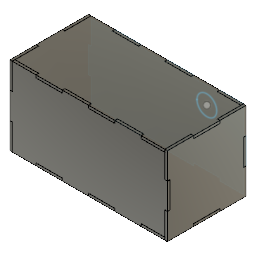
box 4 whole v4 (Autodesk Fusion 360 design; units mm, degrees)
Autodesk Fusion 360 part; units mm, degrees
sketch "Sketch1" plane through (0, 0, 0) normal (0, 0, 1) x (1, 0, 0)
  line L0 (0, 0) -> (120, 0)
  line L1 (120, 0) -> (120, 60)
  line L2 (120, 60) -> (0, 60)
  line L3 (0, 60) -> (0, 0)
  line L4 (0, 60) -> (20, 60)
  line L5 (20, 60) -> (20, 58)
  line L6 (20, 58) -> (0, 58)
  line L7 (0, 58) -> (0, 60)
  line L8 (20, 60) -> (40, 60)
  line L9 (40, 60) -> (40, 58)
  line L10 (40, 58) -> (20, 58)
  line L11 (20, 58) -> (20, 60)
  line L12 (40, 60) -> (60, 60)
  line L13 (60, 60) -> (60, 58)
  line L14 (60, 58) -> (40, 58)
  line L15 (40, 58) -> (40, 60)
  line L16 (60, 60) -> (80, 60)
  line L17 (80, 60) -> (80, 58)
  line L18 (80, 58) -> (60, 58)
  line L19 (60, 58) -> (60, 60)
  line L20 (80, 60) -> (100, 60)
  line L21 (100, 60) -> (100, 58)
  line L22 (100, 58) -> (80, 58)
  line L23 (80, 58) -> (80, 60)
  line L24 (100, 60) -> (120, 60)
  line L25 (120, 60) -> (120, 58)
  line L26 (120, 58) -> (100, 58)
  line L27 (100, 58) -> (100, 60)
  line L28 (120, 60) -> (118, 60)
  line L29 (118, 60) -> (118, 40)
  line L30 (118, 40) -> (120, 40)
  line L31 (120, 40) -> (120, 60)
  line L32 (118, 40) -> (120, 40)
  line L33 (120, 40) -> (120, 20)
  line L34 (120, 20) -> (118, 20)
  line L35 (118, 20) -> (118, 40)
  line L36 (120, 20) -> (118, 20)
  line L37 (118, 20) -> (118, 0)
  line L38 (118, 0) -> (120, 0)
  line L39 (120, 0) -> (120, 20)
  line L40 (120, 0) -> (100, 0)
  line L41 (100, 0) -> (100, 2)
  line L42 (100, 2) -> (120, 2)
  line L43 (120, 2) -> (120, 0)
  line L44 (100, 2) -> (80, 2)
  line L45 (80, 2) -> (80, 0)
  line L46 (80, 0) -> (100, 0)
  line L47 (100, 0) -> (100, 2)
  line L48 (80, 2) -> (60, 2)
  line L49 (60, 2) -> (60, 0)
  line L50 (60, 0) -> (80, 0)
  line L51 (80, 0) -> (80, 2)
  line L52 (60, 2) -> (40, 2)
  line L53 (40, 2) -> (40, 0)
  line L54 (40, 0) -> (60, 0)
  line L55 (60, 0) -> (60, 2)
  line L56 (40, 2) -> (20, 2)
  line L57 (20, 2) -> (20, 0)
  line L58 (20, 0) -> (40, 0)
  line L59 (40, 0) -> (40, 2)
  line L60 (20, 2) -> (0, 2)
  line L61 (0, 2) -> (0, 0)
  line L62 (0, 0) -> (20, 0)
  line L63 (20, 0) -> (20, 2)
  line L64 (0, 0) -> (2, 0)
  line L65 (2, 0) -> (2, 20)
  line L66 (2, 20) -> (0, 20)
  line L67 (0, 20) -> (0, 0)
  line L68 (0, 20) -> (2, 20)
  line L69 (2, 20) -> (2, 40)
  line L70 (2, 40) -> (0, 40)
  line L71 (0, 40) -> (0, 20)
  line L72 (0, 40) -> (2, 40)
  line L73 (2, 40) -> (2, 60)
  line L74 (2, 60) -> (0, 60)
  line L75 (0, 60) -> (0, 40)
  dimension "d1" = 120
  dimension "d2" = 60
  dimension "d3" = 20
  dimension "d4" = 2
  dimension "d5" = 20
  dimension "d6" = 2
  dimension "d7" = 20
  dimension "d8" = 2
  dimension "d9" = 20
  dimension "d10" = 2
  dimension "d11" = 20
  dimension "d12" = 2
  dimension "d13" = 20
  dimension "d14" = 2
  dimension "d15" = 2
  dimension "d16" = 20
  dimension "d17" = 2
  dimension "d18" = 20
  dimension "d19" = 2
  dimension "d20" = 20
  dimension "d21" = 20
  dimension "d22" = 2
  dimension "d23" = 20
  dimension "d24" = 2
  dimension "d25" = 20
  dimension "d26" = 2
  dimension "d27" = 20
  dimension "d28" = 2
  dimension "d29" = 20
  dimension "d30" = 2
  dimension "d31" = 20
  dimension "d32" = 2
  dimension "d33" = 2
  dimension "d34" = 20
  dimension "d35" = 2
  dimension "d36" = 20
  dimension "d37" = 2
  dimension "d38" = 20
  constraint horizontal L0
  constraint vertical L1
  constraint horizontal L2
  constraint vertical L3
  constraint coincident L0.start L3.end
  constraint horizontal L4
  constraint vertical L5
  constraint horizontal L6
  constraint vertical L7
  constraint horizontal L8
  constraint vertical L9
  constraint horizontal L10
  constraint vertical L11
  constraint horizontal L12
  constraint vertical L13
  constraint horizontal L14
  constraint vertical L15
  constraint horizontal L16
  constraint vertical L17
  constraint horizontal L18
  constraint vertical L19
  constraint horizontal L20
  constraint vertical L21
  constraint horizontal L22
  constraint vertical L23
  constraint horizontal L24
  constraint vertical L25
  constraint horizontal L26
  constraint vertical L27
  constraint horizontal L28
  constraint vertical L29
  constraint horizontal L30
  constraint vertical L31
  constraint horizontal L32
  constraint vertical L33
  constraint horizontal L34
  constraint vertical L35
  constraint horizontal L36
  constraint vertical L37
  constraint horizontal L38
  constraint vertical L39
  constraint horizontal L40
  constraint vertical L41
  constraint horizontal L42
  constraint vertical L43
  constraint horizontal L44
  constraint vertical L45
  constraint horizontal L46
  constraint vertical L47
  constraint horizontal L48
  constraint vertical L49
  constraint horizontal L50
  constraint vertical L51
  constraint horizontal L52
  constraint vertical L53
  constraint horizontal L54
  constraint vertical L55
  constraint horizontal L56
  constraint vertical L57
  constraint horizontal L58
  constraint vertical L59
  constraint horizontal L60
  constraint vertical L61
  constraint horizontal L62
  constraint vertical L63
  constraint horizontal L64
  constraint vertical L65
  constraint horizontal L66
  constraint vertical L67
  constraint horizontal L68
  constraint vertical L69
  constraint horizontal L70
  constraint vertical L71
  constraint horizontal L72
  constraint vertical L73
  constraint horizontal L74
  constraint vertical L75
  measures "d1" distance of L0.start L0.end
  measures "d2" distance of L0.start L2.end
  measures "d3" distance of L2.end L4.end
  measures "d4" distance of L2.end L6.end
  measures "d5" distance of L4.end L8.end
  measures "d6" distance of L4.end L5.end
  measures "d7" distance of L8.end L12.end
  measures "d8" distance of L8.end L9.end
  measures "d9" distance of L12.end L16.end
  measures "d10" distance of L12.end L13.end
  measures "d11" distance of L16.end L20.end
  measures "d12" distance of L16.end L17.end
  measures "d13" distance of L20.end L1.end
  measures "d14" distance of L20.end L21.end
  measures "d15" distance of L1.end L28.end
  measures "d16" distance of L1.end L30.end
  measures "d17" distance of L29.end L30.end
  measures "d18" distance of L29.end L34.end
  measures "d19" distance of L33.end L34.end
  measures "d20" distance of L33.end L0.end
  measures "d21" distance of L0.end L40.end
  measures "d22" distance of L0.end L42.end
  measures "d23" distance of L41.end L44.end
  measures "d24" distance of L41.end L40.end
  measures "d25" distance of L44.end L48.end
  measures "d26" distance of L44.end L45.end
  measures "d27" distance of L48.end L52.end
  measures "d28" distance of L48.end L49.end
  measures "d29" distance of L52.end L56.end
  measures "d30" distance of L52.end L53.end
  measures "d31" distance of L56.end L60.end
  measures "d32" distance of L56.end L57.end
  measures "d33" distance of L0.start L64.end
  measures "d34" distance of L0.start L66.end
  measures "d35" distance of L66.end L65.end
  measures "d36" distance of L66.end L70.end
  measures "d37" distance of L70.end L69.end
  measures "d38" distance of L70.end L2.end
extrude "Extrude1" add sketch "Sketch1" along normal blind 2 contours L0 L53 L56 L57 L58 L59 L63 | L6 L10 L14 L18 L22 L26 L29 L35 L37 L42 L44 L48 L52 L56 L60 L65 L69 L73 | L3 L66 L68 L69 L70 L71 L72 | L0 L45 L48 L49 L50 L51 L55 | L2 L4 L5 L6 L11 L73 | L0 L37 L40 L41 L42 L47 | L2 L9 L12 L13 L14 L15 L19 | L1 L30 L32 L33 L34 L35 L36 | L2 L17 L20 L21 L22 L23 L27 makes body 1
sketch "Sketch2" plane through (0, 0, 0) normal (1, 0, 0) x (0, 1, 0)
  line L0 (0, 0) -> (60, 0)
  line L1 (60, 0) -> (60, 60)
  line L2 (60, 60) -> (0, 60)
  line L3 (0, 60) -> (0, 0)
  line L4 (60, 0) -> (40, 0)
  line L5 (40, 0) -> (40, 2)
  line L6 (40, 2) -> (60, 2)
  line L7 (60, 2) -> (60, 0)
  line L8 (0, 0) -> (20, 0)
  line L9 (20, 0) -> (20, 2)
  line L10 (20, 2) -> (0, 2)
  line L11 (0, 2) -> (0, 0)
  line L12 (0, 60) -> (2, 60)
  line L13 (2, 60) -> (2, 40)
  line L14 (2, 40) -> (0, 40)
  line L15 (0, 40) -> (0, 60)
  line L16 (2, 40) -> (0, 40)
  line L17 (0, 40) -> (0, 20)
  line L18 (0, 20) -> (2, 20)
  line L19 (2, 20) -> (2, 40)
  line L20 (0, 20) -> (2, 20)
  line L21 (2, 20) -> (2, 0)
  line L22 (2, 0) -> (0, 0)
  line L23 (0, 0) -> (0, 20)
  line L24 (60, 60) -> (58, 60)
  line L25 (58, 60) -> (58, 40)
  line L26 (58, 40) -> (60, 40)
  line L27 (60, 40) -> (60, 60)
  line L28 (58, 40) -> (60, 40)
  line L29 (60, 40) -> (60, 20)
  line L30 (60, 20) -> (58, 20)
  line L31 (58, 20) -> (58, 40)
  line L32 (60, 20.0791) -> (58, 20.0791)
  line L33 (58, 20.0791) -> (58, 0)
  line L34 (58, 0) -> (60, 0)
  line L35 (60, 0) -> (60, 20.0791)
  line L36 (60, 60) -> (40, 60)
  line L37 (40, 60) -> (40, 58)
  line L38 (40, 58) -> (60, 58)
  line L39 (60, 58) -> (60, 60)
  line L40 (40, 60) -> (20, 60)
  line L41 (20, 60) -> (20, 58)
  line L42 (20, 58) -> (40, 58)
  line L43 (40, 58) -> (40, 60)
  line L44 (20, 60) -> (0, 60)
  line L45 (0, 60) -> (0, 58)
  line L46 (0, 58) -> (20, 58)
  line L47 (20, 58) -> (20, 60)
  line L48 (40, 2) -> (20, 2)
  line L49 (20, 2) -> (20, 0)
  line L50 (20, 0) -> (40, 0)
  line L51 (40, 0) -> (40, 2)
  dimension "d41" = 60
  dimension "d42" = 60
  constraint horizontal L0
  constraint vertical L1
  constraint horizontal L2
  constraint vertical L3
  constraint coincident L0.start L3.end
  constraint horizontal L4
  constraint vertical L5
  constraint horizontal L6
  constraint vertical L7
  constraint horizontal L8
  constraint vertical L9
  constraint horizontal L10
  constraint vertical L11
  constraint horizontal L12
  constraint vertical L13
  constraint horizontal L14
  constraint vertical L15
  constraint horizontal L16
  constraint vertical L17
  constraint horizontal L18
  constraint vertical L19
  constraint coincident L3 L17.end
  constraint horizontal L20
  constraint vertical L21
  constraint horizontal L22
  constraint vertical L23
  constraint horizontal L24
  constraint vertical L25
  constraint horizontal L26
  constraint vertical L27
  constraint horizontal L28
  constraint vertical L29
  constraint horizontal L30
  constraint vertical L31
  constraint coincident L1 L29.end
  constraint horizontal L32
  constraint vertical L33
  constraint horizontal L34
  constraint vertical L35
  constraint coincident L4 L33.end
  constraint coincident L1 L32.start
  constraint horizontal L36
  constraint vertical L37
  constraint horizontal L38
  constraint vertical L39
  constraint horizontal L40
  constraint vertical L41
  constraint horizontal L42
  constraint vertical L43
  constraint horizontal L44
  constraint vertical L45
  constraint horizontal L46
  constraint vertical L47
  constraint coincident L15 L45.end
  constraint horizontal L48
  constraint vertical L49
  constraint horizontal L50
  constraint vertical L51
  measures "d41" distance of L0.start L0.end
  measures "d42" distance of L0.start L2.end
extrude "Extrude2" add sketch "Sketch2" along normal blind 2 separate body contours L0 L3 L8 L10 L11 L21 L22 L23 | L0 L8 L9 L10 L21 L49 | L3 L10 L18 L20 L21 L23 | L6 L10 L13 L19 L21 L25 L31 L33 L38 L42 L46 L48 | L0 L4 L5 L6 L33 L51 | L3 L13 L14 L15 L16 L46 | L0 L1 L4 L6 L7 L33 L34 L35 | L2 L3 L12 L13 L15 L44 L45 L46 | L1 L6 L30 L33 L35 | L2 L13 L41 L44 L46 L47 | L2 L25 L36 L37 L38 L43 | L1 L25 L26 L27 L28 L38 | L1 L2 L24 L25 L27 L36 L38 L39 makes body 2
ref_plane "WorkPlane1" through (61, 30, 30) normal (1, 0, 0) x (0, 0, -1)
mirror "Mirror1" about plane through (61, 30, 30) normal (1, 0, 0) of bodies 2 makes body 3
move_body "Move1" bodies 3 to x (1, 0, 0) y (0, 1, 0) z (0, 0, 1) at (-2, 0, 0)
ref_plane "WorkPlane2" through (60, 30, 31) normal (0, 0, 1) x (1, 0, 0)
mirror "Mirror2" about plane through (60, 30, 31) normal (0, 0, 1) of bodies 1 makes body 4
move_body "Move2" bodies 4 to x (1, 0, 0) y (0, 1, 0) z (0, 0, 1) at (0, 0, -2)
sketch "Sketch3" plane through (0, 0, 0) normal (0, 1, 0) x (1, 0, 0)
  line L0 (0, 0) -> (120, 0)
  line L1 (120, 0) -> (120, -60)
  line L2 (120, -60) -> (0, -60)
  line L3 (0, -60) -> (0, 0)
  line L4 (0, -60) -> (2, -60)
  line L5 (2, -60) -> (2, -40)
  line L6 (2, -40) -> (0, -40)
  line L7 (0, -40) -> (0, -60)
  line L8 (0, -40) -> (2, -40)
  line L9 (2, -40) -> (2, -20)
  line L10 (2, -20) -> (0, -20)
  line L11 (0, -20) -> (0, -40)
  line L12 (0, -20) -> (2, -20)
  line L13 (2, -20) -> (2, 0)
  line L14 (2, 0) -> (0, 0)
  line L15 (0, 0) -> (0, -20)
  line L16 (0, -60) -> (20, -60)
  line L17 (20, -60) -> (20, -58)
  line L18 (20, -58) -> (0, -58)
  line L19 (0, -58) -> (0, -60)
  line L20 (20, -60) -> (40, -60)
  line L21 (40, -60) -> (40, -58)
  line L22 (40, -58) -> (20, -58)
  line L23 (20, -58) -> (20, -60)
  line L24 (40, -60) -> (60, -60)
  line L25 (60, -60) -> (60, -58)
  line L26 (60, -58) -> (40, -58)
  line L27 (40, -58) -> (40, -60)
  line L28 (60, -60) -> (80, -60)
  line L29 (80, -60) -> (80, -58)
  line L30 (80, -58) -> (60, -58)
  line L31 (60, -58) -> (60, -60)
  line L32 (80, -60) -> (100, -60)
  line L33 (100, -60) -> (100, -58)
  line L34 (100, -58) -> (80, -58)
  line L35 (80, -58) -> (80, -60)
  line L36 (100, -60) -> (120, -60)
  line L37 (120, -60) -> (120, -58)
  line L38 (120, -58) -> (100, -58)
  line L39 (100, -58) -> (100, -60)
  line L40 (120, -60) -> (118, -60)
  line L41 (118, -60) -> (118, -40)
  line L42 (118, -40) -> (120, -40)
  line L43 (120, -40) -> (120, -60)
  line L44 (120, -40) -> (118, -40)
  line L45 (118, -40) -> (118, -20)
  line L46 (118, -20) -> (120, -20)
  line L47 (120, -20) -> (120, -40)
  line L48 (118, -20) -> (120, -20)
  line L49 (120, -20) -> (120, 0)
  line L50 (120, 0) -> (118, 0)
  line L51 (118, 0) -> (118, -20)
  line L52 (120, 0) -> (100, 0)
  line L53 (100, 0) -> (100, -2)
  line L54 (100, -2) -> (120, -2)
  line L55 (120, -2) -> (120, 0)
  line L56 (100, 0) -> (80, 0)
  line L57 (80, 0) -> (80, -2)
  line L58 (80, -2) -> (100, -2)
  line L59 (100, -2) -> (100, 0)
  line L60 (80, 0) -> (60, 0)
  line L61 (60, 0) -> (60, -2)
  line L62 (60, -2) -> (80, -2)
  line L63 (80, -2) -> (80, 0)
  line L64 (0, 0) -> (20, 0)
  line L65 (20, 0) -> (20, -2)
  line L66 (20, -2) -> (0, -2)
  line L67 (0, -2) -> (0, 0)
  line L68 (40, 0) -> (20, 0)
  line L69 (20, 0) -> (20, -2)
  line L70 (20, -2) -> (40, -2)
  line L71 (40, -2) -> (40, 0)
  line L72 (40, 0) -> (60, 0)
  line L73 (60, 0) -> (60, -2)
  line L74 (60, -2) -> (40, -2)
  line L75 (40, -2) -> (40, 0)
  constraint horizontal L0
  constraint vertical L1
  constraint horizontal L2
  constraint vertical L3
  constraint coincident L0.start L3.end
  constraint horizontal L4
  constraint vertical L5
  constraint horizontal L6
  constraint vertical L7
  constraint horizontal L8
  constraint vertical L9
  constraint horizontal L10
  constraint vertical L11
  constraint horizontal L12
  constraint vertical L13
  constraint horizontal L14
  constraint vertical L15
  constraint coincident L0 L13.end
  constraint horizontal L16
  constraint vertical L17
  constraint horizontal L18
  constraint vertical L19
  constraint horizontal L20
  constraint vertical L21
  constraint horizontal L22
  constraint vertical L23
  constraint horizontal L24
  constraint vertical L25
  constraint horizontal L26
  constraint vertical L27
  constraint horizontal L28
  constraint vertical L29
  constraint horizontal L30
  constraint vertical L31
  constraint horizontal L32
  constraint vertical L33
  constraint horizontal L34
  constraint vertical L35
  constraint horizontal L36
  constraint vertical L37
  constraint horizontal L38
  constraint vertical L39
  constraint coincident L1 L37.end
  constraint horizontal L40
  constraint vertical L41
  constraint horizontal L42
  constraint vertical L43
  constraint horizontal L44
  constraint vertical L45
  constraint horizontal L46
  constraint vertical L47
  constraint horizontal L48
  constraint vertical L49
  constraint horizontal L50
  constraint vertical L51
  constraint horizontal L52
  constraint vertical L53
  constraint horizontal L54
  constraint vertical L55
  constraint horizontal L56
  constraint vertical L57
  constraint horizontal L58
  constraint vertical L59
  constraint horizontal L60
  constraint vertical L61
  constraint horizontal L62
  constraint vertical L63
  constraint horizontal L64
  constraint vertical L65
  constraint horizontal L66
  constraint vertical L67
  constraint horizontal L68
  constraint vertical L69
  constraint horizontal L70
  constraint vertical L71
  constraint coincident L0 L68.start
  constraint horizontal L72
  constraint vertical L73
  constraint horizontal L74
  constraint vertical L75
extrude "Extrude3" add sketch "Sketch3" along normal blind 2 separate body contours L0 L13 L64 L65 L66 L69 | L5 L9 L13 L18 L22 L26 L30 L34 L38 L41 L45 L51 L54 L58 L62 L66 L70 L74 | L3 L6 L8 L9 L10 L11 L12 | L0 L61 L71 L72 L73 L74 L75 | L0 L53 L56 L57 L58 L59 L63 | L2 L5 L16 L17 L18 L23 | L2 L21 L24 L25 L26 L27 L31 | L1 L42 L44 L45 L46 L47 L48 | L2 L29 L32 L33 L34 L35 L39 makes body 5
sketch "Sketch4" plane through (0, 58, 0) normal (0, 1, 0) x (-1, 0, 0)
  line L0 (-118, 0) -> (-100, 0)
  line L1 (-100, 0) -> (-100, 2)
  line L2 (-100, 2) -> (-118, 2)
  line L3 (-118, 2) -> (-118, 0)
  line L4 (-120, 0) -> (0, 0)
  line L5 (0, 0) -> (0, 60)
  line L6 (0, 60) -> (-120, 60)
  line L7 (-120, 60) -> (-120, 0)
  line L8 (-120, 60) -> (-118, 60)
  line L9 (-118, 60) -> (-118, 40)
  line L10 (-118, 40) -> (-120, 40)
  line L11 (-120, 40) -> (-120, 60)
  line L12 (-118, 40) -> (-120, 40)
  line L13 (-120, 40) -> (-120, 20)
  line L14 (-120, 20) -> (-118, 20)
  line L15 (-118, 20) -> (-118, 40)
  line L16 (-120, 20) -> (-118, 20)
  line L17 (-118, 20) -> (-118, 0)
  line L18 (-118, 0) -> (-120, 0)
  line L19 (-120, 0) -> (-120, 20)
  line L20 (-120, 60) -> (-100, 60)
  line L21 (-100, 60) -> (-100, 58)
  line L22 (-100, 58) -> (-120, 58)
  line L23 (-120, 58) -> (-120, 60)
  line L24 (-100, 60) -> (-80, 60)
  line L25 (-80, 60) -> (-80, 58)
  line L26 (-80, 58) -> (-100, 58)
  line L27 (-100, 58) -> (-100, 60)
  line L28 (-80, 60) -> (-60, 60)
  line L29 (-60, 60) -> (-60, 58)
  line L30 (-60, 58) -> (-80, 58)
  line L31 (-80, 58) -> (-80, 60)
  line L32 (-60, 60) -> (-40, 60)
  line L33 (-40, 60) -> (-40, 58)
  line L34 (-40, 58) -> (-60, 58)
  line L35 (-60, 58) -> (-60, 60)
  line L36 (-40, 60) -> (-20, 60)
  line L37 (-20, 60) -> (-20, 58)
  line L38 (-20, 58) -> (-40, 58)
  line L39 (-40, 58) -> (-40, 60)
  line L40 (-20, 60) -> (0, 60)
  line L41 (0, 60) -> (0, 58)
  line L42 (0, 58) -> (-20, 58)
  line L43 (-20, 58) -> (-20, 60)
  line L44 (0, 60) -> (-2, 60)
  line L45 (-2, 60) -> (-2, 40)
  line L46 (-2, 40) -> (0, 40)
  line L47 (0, 40) -> (0, 60)
  line L48 (-2, 40) -> (0, 40)
  line L49 (0, 40) -> (0, 20)
  line L50 (0, 20) -> (-2, 20)
  line L51 (-2, 20) -> (-2, 40)
  line L52 (0, 20) -> (-2, 20)
  line L53 (-2, 20) -> (-2, 0)
  line L54 (-2, 0) -> (0, 0)
  line L55 (0, 0) -> (0, 20)
  line L56 (0, 0) -> (-20, 0)
  line L57 (-20, 0) -> (-20, 2)
  line L58 (-20, 2) -> (0, 2)
  line L59 (0, 2) -> (0, 0)
  line L60 (-20, 2) -> (-40, 2)
  line L61 (-40, 2) -> (-40, 0)
  line L62 (-40, 0) -> (-20, 0)
  line L63 (-20, 0) -> (-20, 2)
  line L64 (-40, 0) -> (-60, 0)
  line L65 (-60, 0) -> (-60, 2)
  line L66 (-60, 2) -> (-40, 2)
  line L67 (-40, 2) -> (-40, 0)
  line L68 (-60, 0) -> (-80, 0)
  line L69 (-80, 0) -> (-80, 2)
  line L70 (-80, 2) -> (-60, 2)
  line L71 (-60, 2) -> (-60, 0)
  line L72 (-80, 0) -> (-100, 0)
  line L73 (-100, 0) -> (-100, 2)
  line L74 (-100, 2) -> (-80, 2)
  line L75 (-80, 2) -> (-80, 0)
  line L76 (-100, 0) -> (-120, 0)
  line L77 (-120, 0) -> (-120, 2)
  line L78 (-120, 2) -> (-100, 2)
  line L79 (-100, 2) -> (-100, 0)
  constraint horizontal L4
  constraint vertical L5
  constraint horizontal L6
  constraint vertical L7
  constraint horizontal L8
  constraint vertical L9
  constraint horizontal L10
  constraint vertical L11
  constraint horizontal L12
  constraint vertical L13
  constraint horizontal L14
  constraint vertical L15
  constraint coincident L7 L13.end
  constraint horizontal L16
  constraint vertical L17
  constraint horizontal L18
  constraint vertical L19
  constraint coincident L0.start L3.end
  constraint horizontal L20
  constraint vertical L21
  constraint horizontal L22
  constraint vertical L23
  constraint horizontal L24
  constraint vertical L25
  constraint horizontal L26
  constraint vertical L27
  constraint horizontal L28
  constraint vertical L29
  constraint horizontal L30
  constraint vertical L31
  constraint horizontal L32
  constraint vertical L33
  constraint horizontal L34
  constraint vertical L35
  constraint horizontal L36
  constraint vertical L37
  constraint horizontal L38
  constraint vertical L39
  constraint horizontal L40
  constraint vertical L41
  constraint horizontal L42
  constraint vertical L43
  constraint coincident L5 L41.end
  constraint horizontal L44
  constraint vertical L45
  constraint horizontal L46
  constraint vertical L47
  constraint horizontal L48
  constraint vertical L49
  constraint horizontal L50
  constraint vertical L51
  constraint coincident L5 L49.end
  constraint horizontal L52
  constraint vertical L53
  constraint horizontal L54
  constraint vertical L55
  constraint coincident L4 L53.end
  constraint horizontal L56
  constraint vertical L57
  constraint horizontal L58
  constraint vertical L59
  constraint horizontal L60
  constraint vertical L61
  constraint horizontal L62
  constraint vertical L63
  constraint coincident L4 L61.end
  constraint horizontal L64
  constraint vertical L65
  constraint horizontal L66
  constraint vertical L67
  constraint horizontal L68
  constraint vertical L69
  constraint horizontal L70
  constraint vertical L71
  constraint horizontal L72
  constraint vertical L73
  constraint horizontal L74
  constraint vertical L75
  constraint coincident L1.end L2.start
  constraint horizontal L76
  constraint vertical L77
  constraint horizontal L78
  constraint vertical L79
  constraint coincident L19 L77.end
extrude "Extrude4" add sketch "Sketch4" along normal blind 2 separate body contours L0 L1 L2 L3 L4 L17 L73 L76 L78 L79 | L2 L9 L15 L17 L22 L26 L30 L34 L38 L42 L45 L51 L53 L58 L60 L66 L70 L74 L78 | L4 L65 L68 L69 L70 L71 L75 | L7 L10 L12 L13 L14 L15 L16 | L4 L57 L60 L61 L62 L63 L67 | L6 L9 L20 L21 L22 L27 | L6 L25 L28 L29 L30 L31 L35 | L5 L46 L48 L49 L50 L51 L52 | L6 L33 L36 L37 L38 L39 L43 makes body 6
sketch "Sketch5" plane through (0, 0, 60) normal (0, 0, 1) x (-1, 0, 0)
  line L0 (0, -40) -> (0, -20)
  line L1 (0, -20) -> (-2, -20)
  line L2 (-2, -20) -> (-2, -2)
  line L3 (-2, -2) -> (-20, -2)
  line L4 (-20, -2) -> (-20, 0)
  line L5 (-20, 0) -> (-40, 0)
  line L6 (-40, 0) -> (-40, -2)
  line L7 (-40, -2) -> (-60, -2)
  line L8 (-60, -2) -> (-60, 0)
  line L9 (-60, 0) -> (-80, 0)
  line L10 (-80, 0) -> (-80, -2)
  line L11 (-80, -2) -> (-100, -2)
  line L12 (-100, -2) -> (-100, 0)
  line L13 (-100, 0) -> (-118, 0)
  line L14 (-118, 0) -> (-118, -20)
  line L15 (-118, -20) -> (-120, -20)
  line L16 (-120, -20) -> (-120, -40)
  line L17 (-120, -40) -> (-118, -40)
  line L18 (-118, -40) -> (-118, -58)
  line L19 (-118, -58) -> (-100, -58)
  line L20 (-100, -58) -> (-100, -60)
  line L21 (-100, -60) -> (-80, -60)
  line L22 (-80, -60) -> (-80, -58)
  line L23 (-80, -58) -> (-60, -58)
  line L24 (-60, -58) -> (-60, -60)
  line L25 (-60, -60) -> (-40, -60)
  line L26 (-40, -60) -> (-40, -58)
  line L27 (-40, -58) -> (-20, -58)
  line L28 (-20, -58) -> (-20, -60)
  line L29 (-20, -60) -> (-2, -60)
  line L30 (-2, -60) -> (-2, -40)
  line L31 (-2, -40) -> (0, -40)
  line L32 (0, -30) -> (-120, -30)
  constraint midpoint L0 L32.start
  constraint midpoint L16 L32.end
sketch "Sketch6" plane through (0, 60, 0) normal (0, 1, 0) x (-1, 0, 0)
  line L0 (-80, 2) -> (-80, 0)
  line L1 (-80, 0) -> (-60, 0)
  line L2 (-60, 0) -> (-60, 2)
  line L3 (-60, 2) -> (-40, 2)
  line L4 (-40, 2) -> (-40, 0)
  line L5 (-40, 0) -> (-20, 0)
  line L6 (-20, 0) -> (-20, 2)
  line L7 (-20, 2) -> (-2, 2)
  line L8 (-2, 2) -> (-2, 20)
  line L9 (-2, 20) -> (0, 20)
  line L10 (0, 20) -> (0, 40)
  line L11 (0, 40) -> (-2, 40)
  line L12 (-2, 40) -> (-2, 58)
  line L13 (-2, 58) -> (-20, 58)
  line L14 (-20, 58) -> (-20, 60)
  line L15 (-20, 60) -> (-40, 60)
  line L16 (-40, 60) -> (-40, 58)
  line L17 (-40, 58) -> (-60, 58)
  line L18 (-60, 58) -> (-60, 60)
  line L19 (-60, 60) -> (-80, 60)
  line L20 (-80, 60) -> (-80, 58)
  line L21 (-80, 58) -> (-100, 58)
  line L22 (-100, 58) -> (-100, 60)
  line L23 (-100, 60) -> (-118, 60)
  line L24 (-118, 60) -> (-118, 40)
  line L25 (-118, 40) -> (-120, 40)
  line L26 (-120, 40) -> (-120, 20)
  line L27 (-120, 20) -> (-118, 20)
  line L28 (-118, 20) -> (-118, 0)
  line L29 (-118, 0) -> (-100, 0)
  line L30 (-100, 0) -> (-100, 2)
  line L31 (-100, 2) -> (-80, 2)
  circle A0 centre (-90, 45) radius 7.5
  dimension "d53" = 15
  measures "d53" diameter of A0
extrude "Extrude5" cut sketch "Sketch6" against normal blind 5 contours A0 bodies 6
sketch "Sketch7" plane through (0, 60, 0) normal (0, 1, 0) x (-1, 0, 0)
  circle A0 centre (-90, 45) radius 7.5
  line L0 (-80, 2) -> (-80, 0)
  line L1 (-80, 0) -> (-60, 0)
  line L2 (-60, 0) -> (-60, 2)
  line L3 (-60, 2) -> (-40, 2)
  line L4 (-40, 2) -> (-40, 0)
  line L5 (-40, 0) -> (-20, 0)
  line L6 (-20, 0) -> (-20, 2)
  line L7 (-20, 2) -> (-2, 2)
  line L8 (-2, 2) -> (-2, 20)
  line L9 (-2, 20) -> (0, 20)
  line L10 (0, 20) -> (0, 40)
  line L11 (0, 40) -> (-2, 40)
  line L12 (-2, 40) -> (-2, 58)
  line L13 (-2, 58) -> (-20, 58)
  line L14 (-20, 58) -> (-20, 60)
  line L15 (-20, 60) -> (-40, 60)
  line L16 (-40, 60) -> (-40, 58)
  line L17 (-40, 58) -> (-60, 58)
  line L18 (-60, 58) -> (-60, 60)
  line L19 (-60, 60) -> (-80, 60)
  line L20 (-80, 60) -> (-80, 58)
  line L21 (-80, 58) -> (-100, 58)
  line L22 (-100, 58) -> (-100, 60)
  line L23 (-100, 60) -> (-118, 60)
  line L24 (-118, 60) -> (-118, 40)
  line L25 (-118, 40) -> (-120, 40)
  line L26 (-120, 40) -> (-120, 20)
  line L27 (-120, 20) -> (-118, 20)
  line L28 (-118, 20) -> (-118, 0)
  line L29 (-118, 0) -> (-100, 0)
  line L30 (-100, 0) -> (-100, 2)
  line L31 (-100, 2) -> (-80, 2)
named bodies: "bottom", "left", "right", "top", "front", "back"
